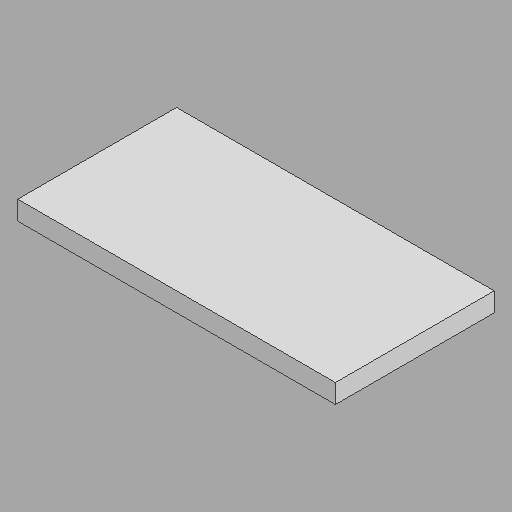
# Autodesk Inventor part: BATTERY_MOUNT_RETROFIT
Saved by Autodesk Inventor 2025.2 (Build 292293000, 293)
## iProperties
Created: 2026-09-05
Part Number: BATTERY_MOUNT_RETROFIT
Material: Generic
Document SubType Name: Modeling
Designer: Ben
Density: 1 g/cm^3
Appearance: Default
Author: Ben
Autodesk Inventor part; units mm, degrees
ref_plane "YZ Plane" through (0, 0, 0) normal (1, 0, 0) x (0, 1, 0)
ref_plane "XZ Plane" through (0, 0, 0) normal (0, 1, 0) x (-1, 0, 0)
ref_plane "XY Plane" through (0, 0, 0) normal (0, 0, 1) x (1, 0, 0)
sketch "Sketch1" plane through (0, 0, 0) normal (0, 0, 1) x (1, 0, 0)
  line L0 (-50, -3) -> (50, -3)
  line L1 (50, -3) -> (50, 3)
  line L2 (50, 3) -> (-50, 3)
  line L3 (-50, 3) -> (-50, -3)
  line L4 (-50, -3) -> (50, 3) construction
  line L5 (50, -3) -> (-50, 3) construction
  point P0 (0, 0)
  dimension "d0" = 6
  dimension "d1" = 100
  constraints: 12 end point, 2 midpoint, 2 parallel, 1 horizontal, 1 perpendicular
  measures "d0" distance of L0.end L1.end
  measures "d1" distance of L1.end L2.end
extrude "Extrusion1" add sketch "Sketch1" along normal mid plane 50
body "Solid1"
